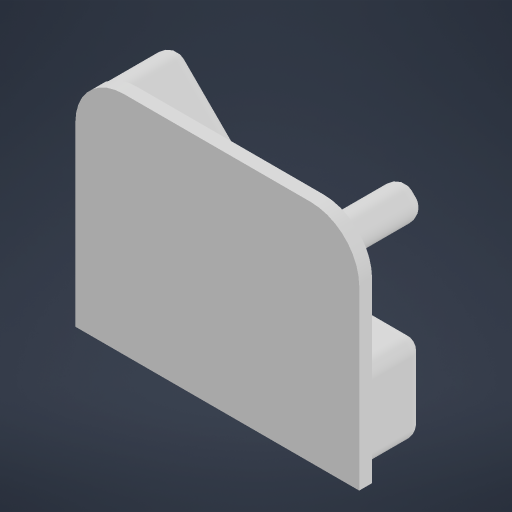
# Autodesk Inventor part: Marker Holder 90 deg
Saved by Autodesk Inventor 2024.1 (Build 281209000, 209)
## iProperties
Created: 2023-09-09
Part Number: Marker Holder 90 deg
Material: Generic
Document SubType Name: Modeling
Designer: User
Density: 1 g/cm^3
Appearance: Default
Author: User
Autodesk Inventor part; units mm, degrees
ref_plane "YZ Plane" through (0, 0, 0) normal (1, 0, 0) x (0, 1, 0)
ref_plane "XZ Plane" through (0, 0, 0) normal (0, 1, 0) x (-1, 0, 0)
ref_plane "XY Plane" through (0, 0, 0) normal (0, 0, 1) x (1, 0, 0)
sketch "Sketch3" plane through (0, 0, 0) normal (0, 0, 1) x (1, 0, 0)
  line L0 (0, 0) -> (40, 0)
  line L1 (40, 0) -> (40, 10)
  line L2 (40, 10) -> (0, 10)
  line L3 (0, 10) -> (0, 0)
  line L4 (20, 10) -> (-1.213203, 31.213203)
  line L5 (-1.213203, 31.213203) -> (2.32233, 34.748737)
  line L6 (2.32233, 34.748737) -> (20, 17.071068)
  line L7 (23.535534, 13.535534) -> (20, 10)
  line L8 (20, 10) -> (50, 10) construction
  line L9 (20, 10) -> (41.213203, 31.213203)
  line L10 (41.213203, 31.213203) -> (37.67767, 34.748737)
  line L11 (37.67767, 34.748737) -> (20, 17.071068)
  line L12 (16.464466, 13.535534) -> (20, 10)
  line L13 (20, 10) -> (50, 10) construction
  line L14 (0, 10) -> (40, 10)
  line L15 (40, 10) -> (40, 13.75)
  line L16 (40, 13.75) -> (0, 13.75)
  line L17 (0, 13.75) -> (0, 10)
  point P0 (23.75, 13.75)
  point P1 (16.25, 13.75)
  dimension "d14" = 40
  dimension "d15" = 10
  dimension "d16" = 30
  dimension "d17" = 135
  dimension "d18" = 5
  dimension "d19" = 45
  dimension "d20" = 5
  dimension "d21" = 3.75
  constraints: 36 end point, 8 parallel, 4 perpendicular, 3 horizontal, 2 equal length, 1 collinear, 1 midpoint
  measures "d14" distance of L2.end L1.end
  measures "d15" distance of L1.end L0.end
  measures "d16" distance of L4.start L4.end
  measures "d17" angle of L8 L4
  measures "d18" distance of L4.end L5.end
  measures "d19" angle of L13 L9
  measures "d20" distance of L10.end L9.end
  measures "d21" distance of L15.end L1.end
extrude "Extrusion3" add sketch "Sketch3" along normal blind 10
fillet "Fillet6" radius 2 22 edges at (11.1612, 25.9099, 0) (7.5184, 22.4816, 0) (28.8388, 25.9099, 0) (32.4816, 22.4816, 0) (8.125, 13.75, 0) (31.875, 13.75, 0) (20, 0, 0) (40, 11.875, 0) (40, 5, 0) (40, 13.75, 5) (40, 0, 5) (0, 13.75, 5) (0, 5, 0) (0, 11.875, 0) (0, 0, 5) (20, 17.0711, 5) (37.6777, 34.7487, 5) (41.2132, 31.2132, 5) (2.3223, 34.7487, 5) (0.5546, 32.981, 0) (-1.2132, 31.2132, 5) (39.4454, 32.981, 0)
sketch "Sketch4" plane through (0, 0, 10) normal (0, 0, 1) x (1, 0, 0)
  arc A0 (39.79899, 29.79899) -> (39.79899, 32.627417) centre (38.384776, 31.213203) ccw
  arc A1 (0.20101, 32.627417) -> (0.20101, 29.79899) centre (1.615224, 31.213203) ccw
  line L0 (-0.384776, 0) -> (40.385224, 0)
  line L1 (40.385224, 0) -> (40.385224, 34)
  line L2 (40.385224, 34) -> (-0.384776, 34)
  line L3 (-0.384776, 34) -> (-0.384776, 0)
  point P0 (0, 0)
  point P1 (40.384776, 0)
  dimension "d26" = 40.77
  dimension "d27" = 34
  constraints: 8 end point, 2 parallel, 1 horizontal, 1 perpendicular
  measures "d26" distance of L2.end L1.end
  measures "d27" distance of L1.end L0.end
extrude "Extrusion4" [suppressed]
sketch "Sketch6" plane through (0, 0, 10) normal (0, 0, 1) x (1, 0, 0)
  line L0 (0, 0) -> (40, 0)
  line L1 (40, 0) -> (40, 35)
  line L2 (40, 35) -> (0, 35)
  line L3 (0, 35) -> (0, 0)
  line L4 (40, 0) -> (42, 0)
  line L5 (42, 0) -> (42, 35)
  line L6 (42, 35) -> (40, 35)
  line L7 (40, 35) -> (40, 0)
  line L8 (0, 35) -> (-2, 35)
  line L9 (-2, 35) -> (-2, 0)
  line L10 (-2, 0) -> (0, 0)
  line L11 (0, 0) -> (0, 35)
  line L12 (-2, 0) -> (42, 0)
  line L13 (42, 0) -> (42, -2)
  line L14 (42, -2) -> (-2, -2)
  line L15 (-2, -2) -> (-2, 0)
  dimension "d36" = 40
  dimension "d37" = 35
  dimension "d38" = 2
  dimension "d39" = 2
  dimension "d40" = 2
  constraints: 32 end point, 8 parallel, 4 horizontal, 4 perpendicular, 2 point on line
  measures "d36" distance of L2.end L1.end
  measures "d37" distance of L1.end L0.end
  measures "d38" distance of L6.end L5.end
  measures "d39" distance of L10.end L9.end
  measures "d40" distance of L12.end L13.end
extrude "Extrusion6" add sketch "Sketch6" along normal blind 2 contours L3 L2 L1 L0 | L10 L9 L8 L3 | L1 L6 L5 L4
fillet "Fillet7" radius 7.5 2 edges at (42, 35, 11) (-2, 35, 11)
body "Solid2"
